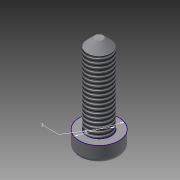
# Autodesk Inventor part: KisLemezcsavar
Saved by Autodesk Inventor 2015 SP1 (Build 190203100, 203)
## iProperties
Created: 2014-11-14
Part Number: KisLemezcsavar
Material: Generic
Document SubType Name: Modeling
Designer: laca
Density: 1 g/cm^3
Appearance: Default
Mass: 0.0961718 g
Surface Area: 1.77257 cm^2
Volume: 0.0961718 cm^3
Author: laca
Autodesk Inventor part; units mm, degrees
ref_plane "YZ Plane" through (0, 0, 0) normal (1, 0, 0) x (0, 1, 0)
ref_plane "XZ Plane" through (0, 0, 0) normal (0, 1, 0) x (-1, 0, 0)
ref_plane "XY Plane" through (0, 0, 0) normal (0, 0, 1) x (1, 0, 0)
sketch "Sketch1" plane through (0, 0, 0) normal (0, 1, 0) x (-1, 0, 0)
  circle A0 centre (0, 0) radius 1.5
  circle A1 centre (0, 0) radius 2.5
  dimension "d0" = 3
  dimension "d1" = 5
  constraints: 2 centre point, 2 coincident
  measures "d0" diameter of A0
  measures "d1" diameter of A1
extrude "Extrusion1" add sketch "Sketch1" along normal blind 10 contours A0
extrude "Extrusion2" add sketch "Sketch1" against normal blind 2 contours A0 | A1
fillet "Fillet1" radius 0.5 1 edges at (2.5, -2, 0)
sketch "Sketch2" plane through (0, -2, 0) normal (0, -1, 0) x (1, 0, 0)
  circle A0 centre (0, 0) radius 1.5 projected
  line L0 (0, 0.5) -> (1.4142, 0.5)
  line L1 (1.4142, 0.5) -> (1.4142, -0.5)
  line L2 (1.4142, -0.5) -> (0, -0.5)
  line L3 (0, -0.5) -> (0, 0.5)
  dimension "d7" = 1
  dimension "d8" = 0.5
  constraints: 8 end point, 2 parallel, 1 horizontal, 1 perpendicular, 2 other
  measures "d7" distance between parallel lines of L2 L0
  measures "d8" distance from line of point (0, 0) L0
extrude "Extrusion3" cut sketch "Sketch2" against normal blind 2 contours L1 L2 L3 L0
pattern_circular "Circular Pattern1" count 4 over 360 about axis through (0, 0, 0) along (0, -1, 0) of "Extrusion3"
thread "Thread1" size "M3x0.5" class "6g" standard "ANSI Metric M Profile" full length
chamfer "Chamfer1" distance 1 angle 45 1 edges at (1.5, 10, 0)
equation "\"d8\" = 0.5 * d7"
body "Solid1"
